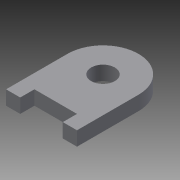
# Autodesk Inventor part: Connector_2
Saved by Autodesk Inventor 2015 (Build 190159000, 159)
## iProperties
Created: 2014-03-20
Part Number: Connector_2
Material: Generic
Document SubType Name: Modeling
Designer: ehagerup
Density: 1 g/cm^3
Appearance: Default
Author: ehagerup
Autodesk Inventor part; units mm, degrees
ref_plane "YZ Plane" through (0, 0, 0) normal (1, 0, 0) x (0, 1, 0)
ref_plane "XZ Plane" through (0, 0, 0) normal (0, 1, 0) x (-1, 0, 0)
ref_plane "XY Plane" through (0, 0, 0) normal (0, 0, 1) x (1, 0, 0)
sketch "Sketch1" plane through (0, 0, 0) normal (0, 0, 1) x (1, 0, 0)
  line L0 (15, 0) -> (15, 13)
  line L1 (0, 13) -> (0, 0)
  arc A0 (15, 13) -> (0, 13) centre (7.5, 13) ccw
  circle A1 centre (7.5, 13) radius 2.5
  line L2 (0, 0) -> (3, 0)
  line L3 (3, 0) -> (3, 3)
  line L4 (0, 3) -> (0, 0)
  line L5 (15, 0) -> (12, 0)
  line L6 (12, 0) -> (12, 3)
  line L7 (15, 3) -> (15, 0)
  line L8 (3, 3) -> (12, 3)
  line L9 (0, 0) -> (3, 0)
  line L10 (12, 0) -> (15, 0)
  dimension "d0" = 15
  dimension "d1" = 13
  dimension "d2" = 5
  constraints: 22 end point, 5 perpendicular, 4 horizontal, 3 parallel, 2 centre point, 2 point on circle, 1 coincident
  measures "d0" distance of L1.start L0.end
  measures "d1" distance of L0.end L0.start
  measures "d2" diameter of A1
extrude "Extrusion1" add sketch "Sketch1" along normal blind 3
body "Solid1"
